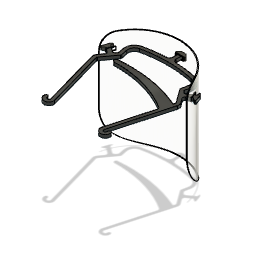
Full_Face_Shield_2 (Autodesk Fusion 360 design; units mm, degrees)
Autodesk Fusion 360 part; units mm, degrees
note: some values were not read from the file. Chosen so that the rebuilt part matches the saved one: which face or edge a step refers to. Set by a fixed rule: which sketch regions a step uses.
sketch "Sketch1" plane through (0, 0, 0) normal (0, 1, 0) x (1, 0, 0)
  line L0 (0, 0) -> (150, 0) construction
  line L1 (150, 0) -> (150, 165) construction
  line L2 (0, 165) -> (0, 0) construction
  line L3 (75, 0) -> (110, 0) construction
  line L4 (75, 0) -> (40, 0) construction
  line L5 (150, 165) -> (150, 115)
  line L6 (0, 165) -> (0, 115) construction
  line L7 (75, 165) -> (15, 165) construction
  line L8 (16.0189, 159.9056) -> (19.5431, 142.2847)
  line L9 (18.5445, 138.1806) -> (1.7256, 117.157)
  line L10 (77.5, 165) -> (135, 165)
  line L11 (133.9811, 159.9056) -> (130.4569, 142.2847)
  line L12 (131.4555, 138.1806) -> (148.2744, 117.157)
  arc A0 (20.1654, 165.8287) -> (16.0189, 159.9056) centre (20.9218, 160.8862) ccw
  arc A1 (133.9811, 159.9056) -> (129.8346, 165.8287) centre (129.0782, 160.8862) ccw
  arc A2 (18.5445, 138.1806) -> (19.5431, 142.2847) centre (14.6402, 141.3041) ccw
  arc A3 (130.4569, 142.2847) -> (131.4555, 138.1806) centre (135.3598, 141.3041) ccw
  arc A4 (1.7256, 117.157) -> (0.9075, 112.391) centre (5.63, 114.0336) ccw
  arc A5 (149.0925, 112.391) -> (148.2744, 117.157) centre (144.37, 114.0336) ccw
  arc A6 (-2.1787, 120.2805) -> (-3.815, 110.7484) centre (5.63, 114.0336) ccw
  line L13 (14.6402, 141.3041) -> (-2.1787, 120.2805)
  line L14 (11.116, 158.925) -> (14.6402, 141.3041)
  arc A7 (19.4091, 170.7711) -> (11.116, 158.925) centre (20.9218, 160.8862) ccw
  arc A8 (130.5909, 170.7711) -> (19.4091, 170.7711) centre (75, -192.5) ccw
  arc A9 (138.884, 158.925) -> (130.5909, 170.7711) centre (129.0782, 160.8862) ccw
  line L15 (138.884, 158.925) -> (135.3598, 141.3041)
  line L16 (135.3598, 141.3041) -> (152.1787, 120.2805)
  arc A10 (153.815, 110.7484) -> (152.1787, 120.2805) centre (144.37, 114.0336) ccw
  line L17 (75, 170) -> (75, 165) construction
  arc A11 (29.827, 93.8884) -> (50.9963, 169.2044) centre (0.8506, 142.666) ccw
  arc A12 (42.1738, 96.8006) -> (56.4371, 169.5244) centre (0.8506, 142.666) ccw
  arc A13 (99.0037, 169.2044) -> (120.173, 93.8884) centre (149.1494, 142.666) ccw
  arc A14 (93.5629, 169.5244) -> (107.8262, 96.8006) centre (149.1494, 142.666) ccw
  circle A15 centre (1.8132, 102.1771) radius 2.5
  circle A16 centre (148.1868, 102.1771) radius 2.5
  line L18 (-3.815, 110.7484) -> (0, 99.7803)
  line L19 (0.9075, 112.391) -> (4.1745, 102.9984)
  line L20 (149.0925, 112.391) -> (145.8255, 102.9984)
  line L21 (153.815, 110.7484) -> (150, 99.7803)
  arc A17 (145.3559, 79.2483) -> (4.6441, 79.2483) centre (75, -70) ccw
  line L22 (-2.88, 72.1259) -> (30, -50)
  arc A18 (30, -50) -> (34.8281, -48.7001) centre (32.414, -49.3501) ccw
  arc A19 (2.5121, 83.771) -> (-2.88, 72.1259) centre (6.7761, 74.7256) ccw
  arc A20 (4.6441, 79.2483) -> (1.948, 73.4257) centre (6.7761, 74.7256) ccw
  line L23 (1.948, 73.4257) -> (34.8281, -48.7001)
  arc A21 (29.827, 93.8884) -> (2.5121, 83.771) centre (75, -70) ccw
  arc A22 (147.4879, 83.771) -> (120.173, 93.8884) centre (75, -70) ccw
  arc A23 (50.9963, 169.2044) -> (20.1654, 165.8287) centre (75, -192.5) ccw
  arc A24 (129.8346, 165.8287) -> (99.0037, 169.2044) centre (75, -192.5) ccw
  line L24 (77.5, 170) -> (77.5, 165)
  line L25 (72.5, 165) -> (72.5, 100)
  line L26 (72.5, 100) -> (72.5, 99.5)
  line L27 (72.5, 99.5) -> (72, 99.5)
  line L28 (72, 99.5) -> (71.8074, 99.5)
  line L29 (77.5, 165) -> (77.5, 99.5)
  line L30 (72.5, 165) -> (72.5, 170.5)
  line L31 (77.5, 169.9914) -> (77.5, 170.5)
  arc A25 (93.5629, 169.5244) -> (77.5, 169.9914) centre (75, -192.5) ccw
  arc A26 (72.5, 169.9914) -> (56.4371, 169.5244) centre (75, -192.5) ccw
  line L32 (150, 165) -> (77.5, 165) construction
  line L33 (75, 165) -> (0, 165) construction
  arc A27 (107.8262, 96.8006) -> (77.5, 99.9816) centre (75, -70) ccw
  arc A28 (72.5, 99.9816) -> (42.1738, 96.8006) centre (75, -70) ccw
  arc A29 (152.88, 72.1259) -> (147.4879, 83.771) centre (143.2239, 74.7256) ccw
  arc A30 (148.052, 73.4257) -> (145.3559, 79.2483) centre (143.2239, 74.7256) ccw
  line L34 (148.052, 73.4257) -> (115.1719, -48.7001)
  line L35 (152.88, 72.1259) -> (120, -50)
  arc A31 (145.3559, 79.2483) -> (4.6441, 79.2483) centre (75, -70) ccw
  arc A32 (115.1719, -48.7001) -> (120, -50) centre (117.586, -49.3501) ccw
  dimension "d1" = 150
  dimension "d2" = 165
  dimension "d3" = 35
  dimension "d4" = 35
  dimension "d5" = 50
  dimension "d6" = 50
  dimension "d7" = 60
  dimension "d8" = 60
  dimension "d9" = 5
  dimension "d14" = 10
  dimension "d15" = -2.5
  constraint horizontal L0
  constraint vertical L1
  constraint horizontal L32
  constraint vertical L2
  constraint coincident L0.start L2.end
  constraint midpoint L0 L3.start
  constraint parallel L0 L3
  constraint parallel L0 L4
  constraint perpendicular L5 L32
  constraint perpendicular L6 L32
  constraint parallel L7 L32
  constraint parallel L10 L32
  constraint coincident L7.end L8
  constraint coincident L7.end A24
  constraint tangent A0 A24
  constraint tangent L8 A0
  constraint coincident L10.end L11
  constraint coincident L10.end A24
  constraint tangent A1 A24
  constraint tangent L11 A1
  constraint equal A0 A1
  constraint tangent L8 A2
  constraint tangent L9 A2
  constraint equal A0 A2
  constraint tangent L11 A3
  constraint tangent L12 A3
  constraint equal A0 A3
  constraint coincident L6.end L9
  constraint coincident L6.end L19
  constraint tangent L9 A4
  constraint tangent A4 L19
  constraint equal A0 A4
  constraint coincident L5.end L12
  constraint coincident L5.end L20
  constraint tangent L12 A5
  constraint tangent A5 L20
  constraint equal A0 A5
  constraint perpendicular L17 L32
  constraint coincident A11.start A22
  constraint coincident A11.end A24
  constraint symmetric L17 A11.end A13.start
  constraint symmetric L17 A11.start A13.end
  constraint symmetric L17 A11 A13
  constraint symmetric L17 A12 A14
  constraint tangent A15 L19
  constraint symmetric L17 A15 A16
  constraint parallel L18 L19
  constraint concentric A4 A6
  constraint parallel L9 L13
  constraint parallel L8 L14
  constraint concentric A0 A7
  constraint concentric A8 A24
  constraint concentric A1 A9
  constraint parallel L11 L15
  constraint parallel L12 L16
  constraint concentric A5 A10
  constraint parallel L20 L21
  constraint tangent A6 L18
  constraint tangent L14 A7
  constraint tangent A7 A8
  constraint tangent A6 L13
  constraint tangent A9 L15
  constraint tangent A8 A9
  constraint tangent L16 A10
  constraint tangent A10 L21
  constraint coincident L2 L18.end
  constraint coincident A15 L19.end
  constraint coincident A16 L20.end
  constraint coincident L1 L21.end
  constraint concentric A17 A22
  constraint tangent A19 A22
  constraint tangent L22 A19
  constraint concentric A11 A12
  constraint concentric A21 A22
  constraint concentric A19 A20
  constraint parallel L22 L23
  constraint tangent A20 L23
  constraint coincident A14.end A22
  constraint concentric A22 A27
  constraint concentric A23 A24
  constraint coincident L17.start A24
  constraint concentric A24 A25
  constraint parallel L25 L26
  constraint perpendicular L26 L27
  constraint perpendicular L26 L28
  constraint perpendicular L27 L29
  constraint parallel L25 L30
  constraint parallel L25 L31
  constraint concentric A25 A26
  constraint coincident L25 A26.start
  constraint collinear L32 L33
  constraint coincident L7.start L32
  constraint coincident L29 A27.end
  constraint coincident L26 A28.start
  constraint concentric A27 A28
  constraint symmetric L17 L22.end L35.end
  constraint symmetric L17 A18.end L34.end
  constraint symmetric L17 L22.start A29.start
  constraint symmetric L17 A19.start A22.start
  constraint symmetric L17 A19 A29
  constraint symmetric L17 A17.end A17.start
  constraint symmetric L17 A20.end A30.start
  constraint symmetric L17 A20 A30
  constraint tangent L35 A32
  measures "d1" distance of L0.start L0.end
  measures "d2" distance of L0.start L2.start
  measures "d3" distance of L3.start L3.end
  measures "d4" distance of L3.start L4.end
  measures "d5" distance of L1.end L5.end
  measures "d6" distance of L2.start L6.end
  measures "d7" distance of L7.start L7.end
  measures "d8" distance of L7.start L10.end
  measures "d9" radius of A0
  measures "d14" radius of A19
sketch "Sketch2" plane through (0, 0, 0) normal (0, 1, 0) x (1, 0, 0)
  arc A0 (74.5, 175.0003) -> (20, 171) centre (74.5, -198.25) ccw
  arc A1 (74.5, 170.0003) -> (20.7301, 166.0536) centre (74.5, -198.25) ccw
  arc A2 (20, 171) -> (11, 159) centre (20.8333, 161) ccw
  line L0 (11, 159) -> (14.1615, 143.4562)
  line L1 (13.1335, 139.2958) -> (-1, 122)
  arc A3 (-1, 122) -> (-3.9689, 110.5533) centre (7.879, 113.5887) ccw
  line L2 (0.3307, 92.0532) -> (30, -50)
  arc A4 (0.3307, 92.0532) -> (-3.9689, 110.5533) centre (-413.7344, 5.5713) ccw
  arc A5 (30, -50) -> (34.8944, -48.9778) centre (32.4472, -49.4889) ccw
  arc A6 (114.1056, -48.9778) -> (119, -50) centre (116.5528, -49.4889) ccw
  arc A7 (13.1335, 139.2958) -> (14.1615, 143.4562) centre (9.2618, 142.4597) ccw
  arc A8 (20.4152, 166.0173) -> (15.8997, 159.9965) centre (20.8333, 161) ccw
  line L3 (15.8997, 159.9965) -> (19.0611, 144.4527)
  arc A9 (17.0052, 136.132) -> (19.0611, 144.4527) centre (9.2618, 142.4597) ccw
  line L4 (17.0052, 136.132) -> (2.7406, 118.6758)
  arc A10 (2.7406, 118.6758) -> (0.8747, 111.7942) centre (7.879, 113.5887) ccw
  arc A11 (5.225, 93.0754) -> (0.8747, 111.7942) centre (-413.7344, 5.5713) ccw
  line L5 (5.225, 93.0754) -> (34.8944, -48.9778)
  line L6 (20.4152, 166.0173) -> (20.7301, 166.0536)
  arc A12 (138, 159) -> (129, 171) centre (128.1667, 161) ccw
  line L7 (133.1003, 159.9965) -> (129.9389, 144.4527)
  line L8 (128.5848, 166.0173) -> (128.2699, 166.0536)
  arc A13 (134.8386, 143.4562) -> (135.8665, 139.2958) centre (139.7382, 142.4597) ccw
  arc A14 (129.9389, 144.4527) -> (131.9948, 136.132) centre (139.7382, 142.4597) ccw
  line L9 (135.8665, 139.2958) -> (150, 122)
  line L10 (138, 159) -> (134.8386, 143.4562)
  arc A15 (129, 171) -> (74.5, 175.0003) centre (74.5, -198.25) ccw
  arc A16 (128.2699, 166.0536) -> (74.5, 170.0003) centre (74.5, -198.25) ccw
  line L11 (131.9948, 136.132) -> (146.2594, 118.6758)
  arc A17 (133.1003, 159.9965) -> (128.5848, 166.0173) centre (128.1667, 161) ccw
  arc A18 (114.1056, -48.9778) -> (119, -50) centre (116.5528, -49.4889) ccw
  arc A19 (148.1253, 111.7942) -> (146.2594, 118.6758) centre (141.121, 113.5887) ccw
  arc A20 (152.9689, 110.5533) -> (148.6693, 92.0532) centre (562.7344, 5.5713) ccw
  line L12 (148.6693, 92.0532) -> (119, -50)
  arc A21 (152.9689, 110.5533) -> (150, 122) centre (141.121, 113.5887) ccw
  arc A22 (141.3302, 87.4373) -> (20, 105) centre (60.9238, -40.1621) ccw
  arc A23 (18.6433, 109.8124) -> (20, 105) centre (19.3216, 107.4062) ccw
  arc A24 (144.5089, 105.6919) -> (38.8673, 114.0893) centre (73.7726, -115.4895) ccw
  arc A25 (143.7795, 100.6741) -> (103.1974, 109.8144) centre (73.7726, -115.4895) ccw
  arc A26 (141.2472, 93.36) -> (103.1974, 109.8144) centre (60.9238, -40.1621) ccw
  arc A27 (38.8673, 114.0893) -> (18.6433, 109.8124) centre (60.9238, -40.1621) ccw
  arc A28 (148.1253, 111.7942) -> (146.9398, 107.0547) centre (562.7344, 5.5713) ccw
  line L13 (142.1794, 85.4361) -> (114.1056, -48.9778)
  arc A29 (144.9419, 98.4876) -> (143.6786, 100.7105) centre (143.0824, 98.9012) ccw
  arc A30 (141.2472, 93.36) -> (144.094, 94.6029) centre (142.2292, 94.9924) ccw
  arc A31 (142.1794, 85.4361) -> (141.3302, 87.4373) centre (140.3146, 85.8256) ccw
  arc A32 (144.5089, 105.6919) -> (146.9398, 107.0547) centre (145.0892, 107.5064) ccw
  line L14 (144.9419, 98.4876) -> (144.094, 94.6029)
  point P0 (149, 0)
  dimension "d17" = -5
  dimension "d18" = 423
  dimension "d19" = -5
  dimension "d20" = 5
  dimension "d23" = 1.905
  dimension "d24" = 1.905
  dimension "d25" = 1.905
  constraint tangent A2 L0
  constraint tangent A3 A4
  constraint tangent L2 A4
  constraint tangent A5 L5
  constraint tangent A22 A23
  constraint concentric A22 A26
  constraint coincident A24.end A26
  constraint concentric A24 A25
  constraint concentric A26 A27
  constraint tangent A26 A30
  constraint equal A29 A30
  constraint tangent A22 A31
  constraint tangent L13 A31
  constraint tangent A24 A32
  constraint tangent A28 A32
  constraint coincident A29 A25.start
  measures "d18" radius of A4
  measures "d20" radius of A7
  measures "d23" radius of A29
  measures "d24" radius of A31
  measures "d25" radius of A32
sketch "Sketch3" plane through (0, 0, 0) normal (0, 1, 0) x (1, 0, 0)
  arc A0 (143.1611, 90.1462) -> (22.4815, 123.2089) centre (28.0682, -93.1729) ccw
  arc A1 (151.4699, 109.6951) -> (21.7483, 130.6442) centre (45.713, -133.0677) ccw
  line L0 (15.076, 155.7601) -> (17.5617, 143.3317)
  line L1 (17.1252, 141.3396) -> (-1.8602, 115.2347)
  line L2 (-2.2518, 113.0551) -> (50.8, -76.2)
  line L3 (75.1061, 175.0001) -> (75.1061, 157.48) construction
  line L4 (135.1363, 155.7601) -> (132.6506, 143.3317)
  line L5 (133.0871, 141.3396) -> (152.0341, 115.2875)
  arc A2 (125.4227, 170.6518) -> (24.7896, 170.6518) centre (75.1061, -57.0962) ccw
  arc A3 (24.7896, 170.6518) -> (15.076, 155.7601) centre (27.5294, 158.2508) ccw
  arc A4 (135.1363, 155.7601) -> (125.4227, 170.6518) centre (122.6829, 158.2508) ccw
  arc A5 (17.1252, 141.3396) -> (17.5617, 143.3317) centre (15.071, 142.8336) ccw
  arc A6 (132.6506, 143.3317) -> (133.0871, 141.3396) centre (135.1413, 142.8336) ccw
  arc A7 (-1.8602, 115.2347) -> (-2.2518, 113.0551) centre (0.1939, 113.7407) ccw
  arc A8 (152.4258, 113.1086) -> (152.0341, 115.2875) centre (149.9799, 113.7935) ccw
  line L6 (-8.3661, 111.3412) -> (44.6857, -77.914)
  arc A9 (-6.9957, 118.9696) -> (-8.3661, 111.3412) centre (0.1939, 113.7407) ccw
  line L7 (8.8493, 154.5148) -> (11.0075, 143.7239)
  arc A10 (23.4197, 176.8522) -> (8.8493, 154.5148) centre (27.5294, 158.2508) ccw
  arc A11 (126.7925, 176.8522) -> (23.4197, 176.8522) centre (75.1061, -57.0962) ccw
  arc A12 (141.363, 154.5148) -> (126.7925, 176.8522) centre (122.6829, 158.2508) ccw
  line L8 (141.363, 154.5148) -> (139.2048, 143.7239)
  arc A13 (158.5406, 111.3962) -> (157.1696, 119.0224) centre (149.9799, 113.7935) ccw
  line L9 (158.5406, 111.3962) -> (105.527, -77.9124)
  arc A14 (99.4123, -76.2) -> (105.527, -77.9124) centre (102.4696, -77.0562) ccw
  arc A15 (44.6857, -77.914) -> (50.8, -76.2) centre (47.7428, -77.057) ccw
  line L10 (152.4258, 113.1086) -> (151.4699, 109.6951)
  line L11 (144.8041, 85.892) -> (99.4123, -76.2)
  arc A16 (10.3842, 0.0056) -> (29.4342, 0.0197) centre (19.9103, -1.4524) ccw
  arc A17 (16.6611, -0.9551) -> (23.1587, -0.9503) centre (19.9103, -1.4524) ccw
  arc A18 (16.6611, -0.9551) -> (10.3842, 0.0056) centre (13.5226, -0.4747) ccw
  arc A19 (120.7781, 0.0197) -> (139.8281, 0.0056) centre (130.302, -1.4524) ccw
  arc A20 (127.0535, -0.9503) -> (133.5512, -0.9551) centre (130.302, -1.4524) ccw
  arc A21 (139.8281, 0.0056) -> (133.5512, -0.9551) centre (136.6896, -0.4747) ccw
  line L12 (120.7781, 0.0197) -> (120.8502, 0.3539)
  line L13 (-13.4671, 150.4121) -> (-17.879, 137.4466)
  line L14 (-1.0754, 133.5877) -> (-10.7402, 140.6166)
  line L15 (-12.1427, 135.7823) -> (-10.7402, 140.6166)
  line L16 (3.1554, 139.4051) -> (-10.0906, 149.0386)
  line L17 (-8.5671, 153.5158) -> (-10.0906, 149.0386)
  line L18 (-17.879, 137.4466) -> (-12.1427, 135.7823)
  line L19 (-8.5671, 153.5158) -> (-10.2135, 154.0761)
  line L20 (11.0075, 143.7239) -> (8.4776, 140.2454)
  line L21 (-0.2351, 128.2655) -> (-6.9957, 118.9696)
  arc A22 (-0.2351, 128.2655) -> (-1.0754, 133.5877) centre (-3.3163, 130.5064) ccw
  arc A23 (3.1554, 139.4051) -> (8.4776, 140.2454) centre (5.3964, 142.4864) ccw
  line L22 (-8.5671, 153.5158) -> (-10.2135, 154.0761)
  line L23 (-10.2135, 154.0761) -> (-13.4671, 150.4121)
  arc A24 (23.3191, 130.7822) -> (23.4173, 123.231) centre (22.86, 127) ccw
  arc A25 (141.7346, 140.2454) -> (147.0568, 139.4051) centre (144.8159, 142.4864) ccw
  arc A26 (151.2877, 133.5877) -> (150.4473, 128.2655) centre (153.5286, 130.5064) ccw
  line L24 (151.2877, 133.5877) -> (160.9524, 140.6166)
  line L25 (147.0568, 139.4051) -> (160.3029, 149.0386)
  line L26 (158.7794, 153.5158) -> (160.3029, 149.0386)
  line L27 (168.0912, 137.4466) -> (162.355, 135.7823)
  line L28 (163.6794, 150.4121) -> (168.0912, 137.4466)
  line L29 (162.355, 135.7823) -> (160.9524, 140.6166)
  line L30 (160.4258, 154.0761) -> (163.6794, 150.4121)
  line L31 (158.7794, 153.5158) -> (160.4258, 154.0761)
  line L32 (139.2048, 143.7239) -> (141.7346, 140.2454)
  line L33 (150.4473, 128.2655) -> (157.1696, 119.0224)
  arc A27 (144.8041, 85.892) -> (143.1611, 90.1462) centre (141.1353, 86.9194) ccw
  dimension "d26" = 7.62
  dimension "d27" = 12.7
  dimension "d28" = 2.54
  dimension "d32" = 19.05
  dimension "d33" = -6.35
  dimension "d41" = 3.81
  dimension "d42" = 3.81
  constraint coincident A0.end A24
  constraint coincident A1.end A24
  constraint vertical L3
  constraint symmetric L2.end L3 A14.start
  constraint tangent A2 A3
  constraint tangent L0 A3
  constraint tangent A2 A4
  constraint tangent L4 A4
  constraint equal A3 A4
  constraint tangent L0 A5
  constraint tangent L1 A5
  constraint tangent L4 A6
  constraint tangent L5 A6
  constraint equal A5 A6
  constraint tangent L1 A7
  constraint tangent L2 A7
  constraint equal A5 A7
  constraint tangent L5 A8
  constraint tangent A8 L10
  constraint equal A5 A8
  constraint tangent L2 A15
  constraint collinear L10 L11
  constraint parallel L2 L6
  constraint concentric A7 A9
  constraint parallel L1 L20
  constraint parallel L0 L7
  constraint concentric A3 A10
  constraint concentric A2 A11
  constraint concentric A4 A12
  constraint parallel L4 L8
  constraint parallel L5 L32
  constraint concentric A8 A13
  constraint tangent L7 A10
  constraint tangent A10 A11
  constraint tangent A13 L9
  constraint tangent A11 A12
  constraint tangent A12 L8
  constraint tangent A13 L32
  constraint coincident L2 A16.end
  constraint tangent A17 A18
  constraint symmetric L3 A16.end A19.start
  constraint symmetric L3 A16.start A19.end
  constraint symmetric L3 A16 A19
  constraint symmetric L3 A17.end A20.start
  constraint symmetric L3 A17.start A20.end
  constraint symmetric L3 A17 A20
  constraint symmetric L3 A18 A21
  constraint coincident L11 L12.end
  constraint perpendicular L14 L20
  constraint perpendicular L16 L20
  constraint parallel L13 L17
  constraint perpendicular L15 L18
  constraint perpendicular L17 L19
  constraint collinear L20 L21
  constraint tangent L21 A22
  constraint tangent L14 A22
  constraint tangent L16 A23
  constraint tangent L20 A23
  constraint equal A22 A23
  constraint coincident A0 A24.end
  constraint coincident A1 A24.start
  constraint symmetric L3 L17.start L26.start
  constraint symmetric L3 L13.end L27.start
  constraint symmetric L3 L14.end L24.end
  constraint symmetric L3 L16.end L25.end
  constraint symmetric L3 L15.start L27.end
  constraint symmetric L3 L21.start A26.end
  constraint symmetric L3 L14.start A26.start
  constraint symmetric L3 A22 A26
  constraint symmetric L3 L16.start A25.end
  constraint symmetric L3 L20.end A25.start
  constraint symmetric L3 A23 A25
  constraint symmetric L3 L19.end L30.start
  constraint symmetric L3 L13.start L28.start
  constraint collinear L32 L33
  constraint tangent A0 A27
  constraint tangent L11 A27
  measures "d26" diameter of A24
  measures "d27" radius of A3
  measures "d28" radius of A5
  measures "d32" distance of A16.end A16.start
  measures "d41" radius of A22
  measures "d42" radius of A27
extrude "Extrude1" add sketch "Sketch3" along normal blind 6.223 contours A0 A1 L0 L1 L2 L4 L5 A2 A3 A4 A5 A6 A7 A8 L6 A9 L7 A10 A11 A12 L8 A13 L9 L10 L11 A16 A19 L12 L13 L14 L15 L16 L17 L18 L19 L20 L21 A22 A23 L22 L23 A24 A25 A26 L24 L25 L26 L27 L28 L29 L30 L31 L32 L33 A27 | A1 A24 makes body 1
sketch "Sketch4" plane through (0, 6.223, 0) normal (0, 1, 0) x (-1, 0, 0)
  arc A0 (-143.1611, -90.1462) -> (-22.4815, -123.2089) centre (-28.0682, 93.1729) ccw
  line L0 (-144.8041, -85.892) -> (-120.8502, -0.3539)
  line L1 (-124.7356, 9.3193) -> (-158.5406, -111.3962)
  arc A1 (-158.5406, -111.3962) -> (-157.1696, -119.0224) centre (-149.9799, -113.7935) ccw
  line L2 (-157.1696, -119.0224) -> (-150.4473, -128.2655)
  line L3 (-139.2048, -143.7239) -> (-141.363, -154.5148)
  arc A2 (-141.363, -154.5148) -> (-126.7925, -176.8522) centre (-122.6829, -158.2508) ccw
  arc A3 (-126.7925, -176.8522) -> (-23.4197, -176.8522) centre (-75.1061, 57.0962) ccw
  arc A4 (-23.4197, -176.8522) -> (-8.8493, -154.5148) centre (-27.5294, -158.2508) ccw
  line L4 (-8.8493, -154.5148) -> (-11.0075, -143.7239)
  line L5 (-11.0075, -143.7239) -> (-8.4776, -140.2454)
  arc A5 (6.9957, -118.9696) -> (8.3661, -111.3412) centre (-0.1939, -113.7407) ccw
  line L6 (8.3661, -111.3412) -> (-25.4605, 9.3307)
  line L7 (-29.4342, -0.0197) -> (2.2518, -113.0551)
  arc A6 (1.8602, -115.2347) -> (2.2518, -113.0551) centre (-0.1939, -113.7407) ccw
  line L8 (1.8602, -115.2347) -> (-17.1252, -141.3396)
  arc A7 (-17.1252, -141.3396) -> (-17.5617, -143.3317) centre (-15.071, -142.8336) ccw
  line L9 (-17.5617, -143.3317) -> (-15.076, -155.7601)
  arc A8 (-24.7896, -170.6518) -> (-15.076, -155.7601) centre (-27.5294, -158.2508) ccw
  arc A9 (-125.4227, -170.6518) -> (-24.7896, -170.6518) centre (-75.1061, 57.0962) ccw
  arc A10 (-135.1363, -155.7601) -> (-125.4227, -170.6518) centre (-122.6829, -158.2508) ccw
  line L10 (-135.1363, -155.7601) -> (-132.6506, -143.3317)
  arc A11 (-132.6506, -143.3317) -> (-133.0871, -141.3396) centre (-135.1413, -142.8336) ccw
  line L11 (-133.0871, -141.3396) -> (-152.0341, -115.2875)
  arc A12 (-152.4258, -113.1086) -> (-152.0341, -115.2875) centre (-149.9799, -113.7935) ccw
  line L12 (-152.4258, -113.1086) -> (-151.4699, -109.6951)
  arc A13 (-151.4699, -109.6951) -> (-23.3191, -130.7822) centre (-45.713, 133.0677) ccw
  arc A14 (-23.3191, -130.7822) -> (-22.4815, -123.2089) centre (-22.86, -127) ccw
  arc A15 (-144.8041, -85.892) -> (-143.1611, -90.1462) centre (-141.1353, -86.9194) ccw
  line L13 (-120.8502, -0.3539) -> (-120.7781, -0.0197)
  arc A16 (-120.7781, -0.0197) -> (-124.7356, 9.3193) centre (-130.302, 1.4524) ccw
  arc A17 (-151.2877, -133.5877) -> (-150.4473, -128.2655) centre (-153.5286, -130.5064) ccw
  line L14 (-151.2877, -133.5877) -> (-160.9524, -140.6166)
  line L15 (-160.9524, -140.6166) -> (-162.355, -135.7823)
  line L16 (-162.355, -135.7823) -> (-168.0912, -137.4466)
  line L17 (-168.0912, -137.4466) -> (-163.6794, -150.4121)
  line L18 (-163.6794, -150.4121) -> (-160.4258, -154.0761)
  line L19 (-160.4258, -154.0761) -> (-158.7794, -153.5158)
  line L20 (-158.7794, -153.5158) -> (-160.3029, -149.0386)
  line L21 (-160.3029, -149.0386) -> (-147.0568, -139.4051)
  arc A18 (-141.7346, -140.2454) -> (-147.0568, -139.4051) centre (-144.8159, -142.4864) ccw
  line L22 (-141.7346, -140.2454) -> (-139.2048, -143.7239)
  arc A19 (-3.1554, -139.4051) -> (-8.4776, -140.2454) centre (-5.3964, -142.4864) ccw
  line L23 (-3.1554, -139.4051) -> (10.0906, -149.0386)
  line L24 (10.0906, -149.0386) -> (8.5671, -153.5158)
  line L25 (8.5671, -153.5158) -> (10.2135, -154.0761)
  line L26 (10.2135, -154.0761) -> (13.4671, -150.4121)
  line L27 (13.4671, -150.4121) -> (17.879, -137.4466)
  line L28 (17.879, -137.4466) -> (12.1427, -135.7823)
  line L29 (12.1427, -135.7823) -> (10.7402, -140.6166)
  line L30 (10.7402, -140.6166) -> (1.0754, -133.5877)
  arc A20 (0.2351, -128.2655) -> (1.0754, -133.5877) centre (3.3163, -130.5064) ccw
  line L31 (0.2351, -128.2655) -> (6.9957, -118.9696)
  arc A21 (-25.4605, 9.3307) -> (-29.4342, -0.0197) centre (-19.9103, 1.4524) ccw
sketch "Sketch6" plane through (0, 6.223, 0) normal (0, 1, 0) x (-1, 0, 0)
sketch "Sketch7" plane through (0, 0, 0) normal (0, 1, 0) x (1, 0, 0)
extrude "Extrude2" add sketch "Sketch3" along normal blind 6.096 separate body contours A0 A1 L0 L1 L2 L4 L5 A2 A3 A4 A5 A6 A7 A8 L6 A9 L7 A10 A11 A12 L8 A13 L9 L10 L11 A16 A19 L12 L13 L14 L15 L16 L17 L18 L19 L20 L21 A22 A23 L22 L23 A24 A25 A26 L24 L25 L26 L27 L28 L29 L30 L31 L32 L33 A27 | L9 A19 A20 A21 | L6 A16 A17 A18 makes body 2
sketch "Sketch8" plane through (0, 0, 0) normal (0, -1, 0) x (1, 0, 0)
  arc A0 (139.8281, -0.0056) -> (120.7781, -0.0197) centre (130.302, 1.4524) ccw
  line L0 (120.7781, -0.0197) -> (120.8502, -0.3539)
  line L1 (120.8502, -0.3539) -> (144.8041, -85.892)
  arc A1 (22.4815, -123.2089) -> (143.1611, -90.1462) centre (28.0682, 93.1729) ccw
  arc A2 (22.4815, -123.2089) -> (21.7483, -130.6442) centre (22.86, -127) ccw
  arc A3 (21.7483, -130.6442) -> (151.4699, -109.6951) centre (45.713, 133.0677) ccw
  line L2 (151.4699, -109.6951) -> (152.4258, -113.1086)
  arc A4 (152.0341, -115.2875) -> (152.4258, -113.1086) centre (149.9799, -113.7935) ccw
  line L3 (152.0341, -115.2875) -> (133.0871, -141.3396)
  arc A5 (133.0871, -141.3396) -> (132.6506, -143.3317) centre (135.1413, -142.8336) ccw
  line L4 (132.6506, -143.3317) -> (135.1363, -155.7601)
  arc A6 (125.4227, -170.6518) -> (135.1363, -155.7601) centre (122.6829, -158.2508) ccw
  arc A7 (24.7896, -170.6518) -> (125.4227, -170.6518) centre (75.1061, 57.0962) ccw
  arc A8 (15.076, -155.7601) -> (24.7896, -170.6518) centre (27.5294, -158.2508) ccw
  line L5 (15.076, -155.7601) -> (17.5617, -143.3317)
  arc A9 (17.5617, -143.3317) -> (17.1252, -141.3396) centre (15.071, -142.8336) ccw
  line L6 (17.1252, -141.3396) -> (-1.8602, -115.2347)
  arc A10 (-2.2518, -113.0551) -> (-1.8602, -115.2347) centre (0.1939, -113.7407) ccw
  line L7 (-2.2518, -113.0551) -> (29.4342, -0.0197)
  arc A11 (29.4342, -0.0197) -> (10.3842, -0.0056) centre (19.9103, 1.4524) ccw
  arc A12 (10.3842, -0.0056) -> (16.6611, 0.9551) centre (13.5226, 0.4747) ccw
  arc A13 (23.1898, 1.2301) -> (16.6611, 0.9551) centre (19.9103, 1.4524) ccw
  line L8 (23.1898, 1.2301) -> (-8.3661, -111.3412)
  arc A14 (-8.3661, -111.3412) -> (-6.9957, -118.9696) centre (0.1939, -113.7407) ccw
  line L9 (-6.9957, -118.9696) -> (-0.2351, -128.2655)
  line L10 (11.0075, -143.7239) -> (8.8493, -154.5148)
  arc A15 (8.8493, -154.5148) -> (23.4197, -176.8522) centre (27.5294, -158.2508) ccw
  arc A16 (23.4197, -176.8522) -> (126.7925, -176.8522) centre (75.1061, 57.0962) ccw
  arc A17 (126.7925, -176.8522) -> (141.363, -154.5148) centre (122.6829, -158.2508) ccw
  line L11 (141.363, -154.5148) -> (139.2048, -143.7239)
  line L12 (139.2048, -143.7239) -> (141.7346, -140.2454)
  arc A18 (157.1696, -119.0224) -> (158.5406, -111.3962) centre (149.9799, -113.7935) ccw
  line L13 (158.5406, -111.3962) -> (127.0318, 1.1197)
  arc A19 (133.5512, 0.9551) -> (127.0318, 1.1197) centre (130.302, 1.4524) ccw
  arc A20 (133.5512, 0.9551) -> (139.8281, -0.0056) centre (136.6896, 0.4747) ccw
  arc A21 (143.1611, -90.1462) -> (144.8041, -85.892) centre (141.1353, -86.9194) ccw
  arc A22 (-1.0754, -133.5877) -> (-0.2351, -128.2655) centre (-3.3163, -130.5064) ccw
  line L14 (-1.0754, -133.5877) -> (-10.7402, -140.6166)
  line L15 (-10.7402, -140.6166) -> (-12.1427, -135.7823)
  line L16 (-12.1427, -135.7823) -> (-17.879, -137.4466)
  line L17 (-17.879, -137.4466) -> (-13.4671, -150.4121)
  line L18 (-13.4671, -150.4121) -> (-10.2135, -154.0761)
  line L19 (-10.2135, -154.0761) -> (-8.5671, -153.5158)
  line L20 (-8.5671, -153.5158) -> (-10.0906, -149.0386)
  line L21 (-10.0906, -149.0386) -> (3.1554, -139.4051)
  arc A23 (8.4776, -140.2454) -> (3.1554, -139.4051) centre (5.3964, -142.4864) ccw
  line L22 (8.4776, -140.2454) -> (11.0075, -143.7239)
  arc A24 (147.0568, -139.4051) -> (141.7346, -140.2454) centre (144.8159, -142.4864) ccw
  line L23 (147.0568, -139.4051) -> (160.3029, -149.0386)
  line L24 (160.3029, -149.0386) -> (158.7794, -153.5158)
  line L25 (158.7794, -153.5158) -> (160.4258, -154.0761)
  line L26 (160.4258, -154.0761) -> (163.6794, -150.4121)
  line L27 (163.6794, -150.4121) -> (168.0912, -137.4466)
  line L28 (168.0912, -137.4466) -> (162.355, -135.7823)
  line L29 (162.355, -135.7823) -> (160.9524, -140.6166)
  line L30 (160.9524, -140.6166) -> (151.2877, -133.5877)
  arc A25 (150.4473, -128.2655) -> (151.2877, -133.5877) centre (153.5286, -130.5064) ccw
  line L31 (150.4473, -128.2655) -> (157.1696, -119.0224)
sketch "Sketch9" plane through (0, 0, 0) normal (0, -1, 0) x (1, 0, 0)
sketch "Sketch10" plane through (0, 0, 0) normal (0, -1, 0) x (1, 0, 0)
  arc A0 (139.8281, -0.0056) -> (120.7781, -0.0197) centre (130.302, 1.4524) ccw
  line L0 (120.7781, -0.0197) -> (120.8502, -0.3539)
  line L1 (120.8502, -0.3539) -> (144.8041, -85.892)
  arc A1 (143.1611, -90.1462) -> (144.8041, -85.892) centre (141.1353, -86.9194) ccw
  arc A2 (22.4815, -123.2089) -> (143.1611, -90.1462) centre (28.0682, 93.1729) ccw
  arc A3 (22.4815, -123.2089) -> (21.7483, -130.6442) centre (22.86, -127) ccw
  arc A4 (21.7483, -130.6442) -> (151.4699, -109.6951) centre (45.713, 133.0677) ccw
  line L2 (151.4699, -109.6951) -> (152.4258, -113.1086)
  arc A5 (152.0341, -115.2875) -> (152.4258, -113.1086) centre (149.9799, -113.7935) ccw
  line L3 (152.0341, -115.2875) -> (133.0871, -141.3396)
  arc A6 (133.0871, -141.3396) -> (132.6506, -143.3317) centre (135.1413, -142.8336) ccw
  line L4 (132.6506, -143.3317) -> (135.1363, -155.7601)
  arc A7 (125.4227, -170.6518) -> (135.1363, -155.7601) centre (122.6829, -158.2508) ccw
  arc A8 (24.7896, -170.6518) -> (125.4227, -170.6518) centre (75.1061, 57.0962) ccw
  arc A9 (15.076, -155.7601) -> (24.7896, -170.6518) centre (27.5294, -158.2508) ccw
  line L5 (15.076, -155.7601) -> (17.5617, -143.3317)
  arc A10 (17.5617, -143.3317) -> (17.1252, -141.3396) centre (15.071, -142.8336) ccw
  line L6 (17.1252, -141.3396) -> (-1.8602, -115.2347)
  arc A11 (-2.2518, -113.0551) -> (-1.8602, -115.2347) centre (0.1939, -113.7407) ccw
  line L7 (-2.2518, -113.0551) -> (29.4342, -0.0197)
  arc A12 (29.4342, -0.0197) -> (10.3842, -0.0056) centre (19.9103, 1.4524) ccw
  arc A13 (10.3842, -0.0056) -> (16.6611, 0.9551) centre (13.5226, 0.4747) ccw
  arc A14 (23.1898, 1.2301) -> (16.6611, 0.9551) centre (19.9103, 1.4524) ccw
  line L8 (23.1898, 1.2301) -> (-8.3661, -111.3412)
  arc A15 (-8.3661, -111.3412) -> (-6.9957, -118.9696) centre (0.1939, -113.7407) ccw
  line L9 (-6.9957, -118.9696) -> (-0.2351, -128.2655)
  arc A16 (-1.0754, -133.5877) -> (-0.2351, -128.2655) centre (-3.3163, -130.5064) ccw
  line L10 (-1.0754, -133.5877) -> (-10.7402, -140.6166)
  line L11 (-10.7402, -140.6166) -> (-12.1427, -135.7823)
  line L12 (-12.1427, -135.7823) -> (-17.879, -137.4466)
  line L13 (-17.879, -137.4466) -> (-13.4671, -150.4121)
  line L14 (-13.4671, -150.4121) -> (-10.2135, -154.0761)
  line L15 (-10.2135, -154.0761) -> (-8.5671, -153.5158)
  line L16 (-8.5671, -153.5158) -> (-10.0906, -149.0386)
  line L17 (-10.0906, -149.0386) -> (3.1554, -139.4051)
  arc A17 (8.4776, -140.2454) -> (3.1554, -139.4051) centre (5.3964, -142.4864) ccw
  line L18 (8.4776, -140.2454) -> (11.0075, -143.7239)
  line L19 (11.0075, -143.7239) -> (8.8493, -154.5148)
  arc A18 (8.8493, -154.5148) -> (23.4197, -176.8522) centre (27.5294, -158.2508) ccw
  arc A19 (23.4197, -176.8522) -> (126.7925, -176.8522) centre (75.1061, 57.0962) ccw
  arc A20 (126.7925, -176.8522) -> (141.363, -154.5148) centre (122.6829, -158.2508) ccw
  line L20 (141.363, -154.5148) -> (139.2048, -143.7239)
  line L21 (139.2048, -143.7239) -> (141.7346, -140.2454)
  arc A21 (147.0568, -139.4051) -> (141.7346, -140.2454) centre (144.8159, -142.4864) ccw
  line L22 (147.0568, -139.4051) -> (160.3029, -149.0386)
  line L23 (160.3029, -149.0386) -> (158.7794, -153.5158)
  line L24 (158.7794, -153.5158) -> (160.4258, -154.0761)
  line L25 (160.4258, -154.0761) -> (163.6794, -150.4121)
  line L26 (163.6794, -150.4121) -> (168.0912, -137.4466)
  line L27 (168.0912, -137.4466) -> (162.355, -135.7823)
  line L28 (162.355, -135.7823) -> (160.9524, -140.6166)
  line L29 (160.9524, -140.6166) -> (151.2877, -133.5877)
  arc A22 (150.4473, -128.2655) -> (151.2877, -133.5877) centre (153.5286, -130.5064) ccw
  line L30 (150.4473, -128.2655) -> (157.1696, -119.0224)
  arc A23 (157.1696, -119.0224) -> (158.5406, -111.3962) centre (149.9799, -113.7935) ccw
  line L31 (158.5406, -111.3962) -> (127.0318, 1.1197)
  arc A24 (133.5512, 0.9551) -> (127.0318, 1.1197) centre (130.302, 1.4524) ccw
  arc A25 (133.5512, 0.9551) -> (139.8281, -0.0056) centre (136.6896, 0.4747) ccw
chamfer "Chamfer1" distance 3.81 angle 45 1 edges at (-12.1427, 3.048, -135.7823) on bodies 2
chamfer "Chamfer2" distance 3.81 angle 45 1 edges at (162.355, 3.048, -135.7823) on bodies 2
sketch "Sketch11" plane through (0, 0, 0) normal (0, 0, 1) x (1, 0, 0)
sketch "Sketch12" plane through (0, 6.096, 0) normal (0, 1, 0) x (-1, 0, 0)
  line L0 (-161.2934, -139.4414) -> (-166.0141, -136.844)
  line L1 (-166.0141, -136.844) -> (-168.0912, -137.4466)
  line L2 (-168.0912, -137.4466) -> (-163.6794, -150.4121)
  line L3 (-163.6794, -150.4121) -> (-160.4258, -154.0761)
  line L4 (-160.4258, -154.0761) -> (-158.7794, -153.5158)
  line L5 (-158.7794, -153.5158) -> (-160.3029, -149.0386)
  line L6 (-160.3029, -149.0386) -> (-147.0568, -139.4051)
  arc A0 (-141.7346, -140.2454) -> (-147.0568, -139.4051) centre (-144.8159, -142.4864) ccw
  line L7 (-141.7346, -140.2454) -> (-139.2048, -143.7239)
  line L8 (-139.2048, -143.7239) -> (-141.363, -154.5148)
  arc A1 (-141.363, -154.5148) -> (-126.7925, -176.8522) centre (-122.6829, -158.2508) ccw
  arc A2 (-126.7925, -176.8522) -> (-23.4197, -176.8522) centre (-75.1061, 57.0962) ccw
  arc A3 (-23.4197, -176.8522) -> (-8.8493, -154.5148) centre (-27.5294, -158.2508) ccw
  line L9 (-8.8493, -154.5148) -> (-11.0075, -143.7239)
  line L10 (-11.0075, -143.7239) -> (-8.4776, -140.2454)
  arc A4 (-3.1554, -139.4051) -> (-8.4776, -140.2454) centre (-5.3964, -142.4864) ccw
  line L11 (-3.1554, -139.4051) -> (10.0906, -149.0386)
  line L12 (10.0906, -149.0386) -> (8.5671, -153.5158)
  line L13 (8.5671, -153.5158) -> (10.2135, -154.0761)
  line L14 (10.2135, -154.0761) -> (13.4671, -150.4121)
  line L15 (13.4671, -150.4121) -> (17.879, -137.4466)
  line L16 (17.879, -137.4466) -> (15.8018, -136.844)
  line L17 (15.8018, -136.844) -> (11.0811, -139.4414)
  line L18 (11.0811, -139.4414) -> (10.7402, -140.6166)
  line L19 (10.7402, -140.6166) -> (1.0754, -133.5877)
  arc A5 (0.2351, -128.2655) -> (1.0754, -133.5877) centre (3.3163, -130.5064) ccw
  line L20 (0.2351, -128.2655) -> (6.9957, -118.9696)
  arc A6 (6.9957, -118.9696) -> (8.3661, -111.3412) centre (-0.1939, -113.7407) ccw
  line L21 (8.3661, -111.3412) -> (-23.1898, 1.2301)
  arc A7 (-16.6611, 0.9551) -> (-23.1898, 1.2301) centre (-19.9103, 1.4524) ccw
  arc A8 (-16.6611, 0.9551) -> (-10.3842, -0.0056) centre (-13.5226, 0.4747) ccw
  arc A9 (-10.3842, -0.0056) -> (-29.4342, -0.0197) centre (-19.9103, 1.4524) ccw
  line L22 (-29.4342, -0.0197) -> (2.2518, -113.0551)
  arc A10 (1.8602, -115.2347) -> (2.2518, -113.0551) centre (-0.1939, -113.7407) ccw
  line L23 (1.8602, -115.2347) -> (-17.1252, -141.3396)
  arc A11 (-17.1252, -141.3396) -> (-17.5617, -143.3317) centre (-15.071, -142.8336) ccw
  line L24 (-17.5617, -143.3317) -> (-15.076, -155.7601)
  arc A12 (-24.7896, -170.6518) -> (-15.076, -155.7601) centre (-27.5294, -158.2508) ccw
  arc A13 (-125.4227, -170.6518) -> (-24.7896, -170.6518) centre (-75.1061, 57.0962) ccw
  arc A14 (-135.1363, -155.7601) -> (-125.4227, -170.6518) centre (-122.6829, -158.2508) ccw
  line L25 (-135.1363, -155.7601) -> (-132.6506, -143.3317)
  arc A15 (-132.6506, -143.3317) -> (-133.0871, -141.3396) centre (-135.1413, -142.8336) ccw
  line L26 (-133.0871, -141.3396) -> (-152.0341, -115.2875)
  arc A16 (-152.4258, -113.1086) -> (-152.0341, -115.2875) centre (-149.9799, -113.7935) ccw
  line L27 (-152.4258, -113.1086) -> (-151.4699, -109.6951)
  arc A17 (-151.4699, -109.6951) -> (-21.7483, -130.6442) centre (-45.713, 133.0677) ccw
  arc A18 (-21.7483, -130.6442) -> (-22.4815, -123.2089) centre (-22.86, -127) ccw
  arc A19 (-143.1611, -90.1462) -> (-22.4815, -123.2089) centre (-28.0682, 93.1729) ccw
  arc A20 (-144.8041, -85.892) -> (-143.1611, -90.1462) centre (-141.1353, -86.9194) ccw
  line L28 (-144.8041, -85.892) -> (-120.8502, -0.3539)
  line L29 (-120.8502, -0.3539) -> (-120.7781, -0.0197)
  arc A21 (-120.7781, -0.0197) -> (-139.8281, -0.0056) centre (-130.302, 1.4524) ccw
  arc A22 (-139.8281, -0.0056) -> (-133.5512, 0.9551) centre (-136.6896, 0.4747) ccw
  arc A23 (-127.0318, 1.1197) -> (-133.5512, 0.9551) centre (-130.302, 1.4524) ccw
  line L30 (-127.0318, 1.1197) -> (-158.5406, -111.3962)
  arc A24 (-158.5406, -111.3962) -> (-157.1696, -119.0224) centre (-149.9799, -113.7935) ccw
  line L31 (-157.1696, -119.0224) -> (-150.4473, -128.2655)
  arc A25 (-151.2877, -133.5877) -> (-150.4473, -128.2655) centre (-153.5286, -130.5064) ccw
  line L32 (-151.2877, -133.5877) -> (-160.9524, -140.6166)
  line L33 (-160.9524, -140.6166) -> (-161.2934, -139.4414)
  arc A26 (-160.02, -127) -> (10.16, -127) centre (-74.93, -111.76) ccw
  arc A27 (-161.5826, -127.2799) -> (11.7226, -127.2799) centre (-74.93, -111.76) ccw
  line L34 (11.7226, -127.2799) -> (10.16, -127)
  line L35 (-160.02, -127) -> (-161.5826, -127.2799)
  dimension "d45" = 1.5875
extrude "Extrude3" add sketch "Sketch12" along normal blind 25.4 and the other way blind 177.8 separate body contours L32 A26 A27 L35 | L6 L32 A26 A27 | L6 L11 A26 A27 | L11 L19 A26 A27 | L19 A26 A27 L34 makes body 3
sketch "Sketch13" plane through (0, 0, 0) normal (1, 0, 0) x (0, 0, -1)
  arc A0 (127, -88.9) -> (203.2, -165.1) centre (204.8972, -87.2028) ccw
  line L0 (127, -88.9) -> (114.3, -88.9)
  line L1 (114.3, -88.9) -> (114.3, -177.8)
  line L2 (114.3, -177.8) -> (203.2, -177.8)
  line L3 (203.2, -177.8) -> (203.2, -165.1)
  constraint horizontal L0
  constraint perpendicular L0 L1
  constraint perpendicular L1 L2
extrude "Extrude4" cut sketch "Sketch13" along normal blind -50.8 and the other way blind -292.1 bodies 3
fillet "Fillet1" radius 25.4 2 edges at (-10.9413, 31.496, -127.1399) (160.8013, 31.496, -127.1399) on bodies 3
sketch "Sketch14" plane through (0, 6.096, 0) normal (0, 1, 0) x (-1, 0, 0)
  line L0 (-161.2934, -139.4414) -> (-166.0141, -136.844)
  line L1 (-166.0141, -136.844) -> (-168.0912, -137.4466)
  line L2 (-168.0912, -137.4466) -> (-163.6794, -150.4121)
  line L3 (-163.6794, -150.4121) -> (-160.4258, -154.0761)
  line L4 (-160.4258, -154.0761) -> (-158.7794, -153.5158)
  line L5 (-158.7794, -153.5158) -> (-160.3029, -149.0386)
  line L6 (-160.3029, -149.0386) -> (-147.0568, -139.4051)
  arc A0 (-141.7346, -140.2454) -> (-147.0568, -139.4051) centre (-144.8159, -142.4864) ccw
  line L7 (-141.7346, -140.2454) -> (-139.2048, -143.7239)
  line L8 (-139.2048, -143.7239) -> (-141.363, -154.5148)
  arc A1 (-141.363, -154.5148) -> (-126.7925, -176.8522) centre (-122.6829, -158.2508) ccw
  arc A2 (-126.7925, -176.8522) -> (-23.4197, -176.8522) centre (-75.1061, 57.0962) ccw
  arc A3 (-23.4197, -176.8522) -> (-8.8493, -154.5148) centre (-27.5294, -158.2508) ccw
  line L9 (-8.8493, -154.5148) -> (-11.0075, -143.7239)
  line L10 (-11.0075, -143.7239) -> (-8.4776, -140.2454)
  arc A4 (-3.1554, -139.4051) -> (-8.4776, -140.2454) centre (-5.3964, -142.4864) ccw
  line L11 (-3.1554, -139.4051) -> (10.0906, -149.0386)
  line L12 (10.0906, -149.0386) -> (8.5671, -153.5158)
  line L13 (8.5671, -153.5158) -> (10.2135, -154.0761)
  line L14 (10.2135, -154.0761) -> (13.4671, -150.4121)
  line L15 (13.4671, -150.4121) -> (17.879, -137.4466)
  line L16 (17.879, -137.4466) -> (15.8018, -136.844)
  line L17 (15.8018, -136.844) -> (11.0811, -139.4414)
  line L18 (11.0811, -139.4414) -> (10.7402, -140.6166)
  line L19 (10.7402, -140.6166) -> (1.0754, -133.5877)
  arc A5 (0.2351, -128.2655) -> (1.0754, -133.5877) centre (3.3163, -130.5064) ccw
  line L20 (0.2351, -128.2655) -> (6.9957, -118.9696)
  arc A6 (6.9957, -118.9696) -> (8.3661, -111.3412) centre (-0.1939, -113.7407) ccw
  line L21 (8.3661, -111.3412) -> (-23.1898, 1.2301)
  arc A7 (-16.6611, 0.9551) -> (-23.1898, 1.2301) centre (-19.9103, 1.4524) ccw
  arc A8 (-16.6611, 0.9551) -> (-10.3842, -0.0056) centre (-13.5226, 0.4747) ccw
  arc A9 (-10.3842, -0.0056) -> (-29.4342, -0.0197) centre (-19.9103, 1.4524) ccw
  line L22 (-29.4342, -0.0197) -> (2.2518, -113.0551)
  arc A10 (1.8602, -115.2347) -> (2.2518, -113.0551) centre (-0.1939, -113.7407) ccw
  line L23 (1.8602, -115.2347) -> (-17.1252, -141.3396)
  arc A11 (-17.1252, -141.3396) -> (-17.5617, -143.3317) centre (-15.071, -142.8336) ccw
  line L24 (-17.5617, -143.3317) -> (-15.076, -155.7601)
  arc A12 (-24.7896, -170.6518) -> (-15.076, -155.7601) centre (-27.5294, -158.2508) ccw
  arc A13 (-125.4227, -170.6518) -> (-24.7896, -170.6518) centre (-75.1061, 57.0962) ccw
  arc A14 (-135.1363, -155.7601) -> (-125.4227, -170.6518) centre (-122.6829, -158.2508) ccw
  line L25 (-135.1363, -155.7601) -> (-132.6506, -143.3317)
  arc A15 (-132.6506, -143.3317) -> (-133.0871, -141.3396) centre (-135.1413, -142.8336) ccw
  line L26 (-133.0871, -141.3396) -> (-152.0341, -115.2875)
  arc A16 (-152.4258, -113.1086) -> (-152.0341, -115.2875) centre (-149.9799, -113.7935) ccw
  line L27 (-152.4258, -113.1086) -> (-151.4699, -109.6951)
  arc A17 (-151.4699, -109.6951) -> (-21.7483, -130.6442) centre (-45.713, 133.0677) ccw
  arc A18 (-21.7483, -130.6442) -> (-22.4815, -123.2089) centre (-22.86, -127) ccw
  arc A19 (-143.1611, -90.1462) -> (-22.4815, -123.2089) centre (-28.0682, 93.1729) ccw
  arc A20 (-144.8041, -85.892) -> (-143.1611, -90.1462) centre (-141.1353, -86.9194) ccw
  line L28 (-144.8041, -85.892) -> (-120.8502, -0.3539)
  line L29 (-120.8502, -0.3539) -> (-120.7781, -0.0197)
  arc A21 (-120.7781, -0.0197) -> (-139.8281, -0.0056) centre (-130.302, 1.4524) ccw
  arc A22 (-139.8281, -0.0056) -> (-133.5512, 0.9551) centre (-136.6896, 0.4747) ccw
  arc A23 (-127.0318, 1.1197) -> (-133.5512, 0.9551) centre (-130.302, 1.4524) ccw
  line L30 (-127.0318, 1.1197) -> (-158.5406, -111.3962)
  arc A24 (-158.5406, -111.3962) -> (-157.1696, -119.0224) centre (-149.9799, -113.7935) ccw
  line L31 (-157.1696, -119.0224) -> (-150.4473, -128.2655)
  arc A25 (-151.2877, -133.5877) -> (-150.4473, -128.2655) centre (-153.5286, -130.5064) ccw
  line L32 (-151.2877, -133.5877) -> (-160.9524, -140.6166)
  line L33 (-160.9524, -140.6166) -> (-161.2934, -139.4414)
  arc A26 (-126.7925, -176.8522) -> (-23.4197, -176.8522) centre (-75.1061, 57.0962) ccw
  line L34 (-75.1061, -182.4938) -> (-75.1061, -200.66)
  arc A27 (-85.293, -199.9179) -> (-64.9266, -199.9687) centre (-74.93, -127.9586) ccw
  arc A28 (-84.3528, -206.4466) -> (-65.8656, -206.4888) centre (-74.93, -127.9586) ccw
  line L35 (-78.2811, -182.4938) -> (-78.2811, -200.66)
  line L36 (-71.9311, -182.4938) -> (-71.9311, -200.66)
  line L37 (-65.8656, -206.4888) -> (-64.9266, -199.9687)
  line L38 (-84.3467, -206.4888) -> (-85.2856, -199.9687)
  line L39 (-85.2856, -199.9687) -> (-85.293, -199.9179)
  line L40 (-71.9311, -182.4938) -> (-71.9311, -182.2863)
  line L41 (-71.9311, -182.2863) -> (-78.2877, -182.2863)
  line L42 (-78.2877, -182.2863) -> (-78.2811, -182.4938)
  dimension "d56" = 3.175
  dimension "d57" = -3.175
  constraint coincident A1.end A2.start
  constraint coincident A2.end A3.start
  constraint midpoint A26 L34.start
  constraint vertical L34
  constraint coincident L34.end A27
  constraint symmetric L34 A28.end L38.start
  constraint symmetric L34 A27.end L38.end
  constraint concentric A27 A28
  constraint parallel L38 L39
  constraint coincident L38 A28.start
  constraint parallel L36 L40
  constraint perpendicular L40 L41
extrude "Extrude5" add sketch "Sketch14" against normal blind 6.096 separate body contours A2 A26 L34 A27 L35 L42 | A2 A26 L34 A27 L36 L40 | A27 A28 L37 L38 L39 makes body 4
combine "Combine1" operation add target body 2 tool bodies 4
chamfer "Chamfer3" distance 1.27 angle 45 2 edges at (64.9266, 3.048, -199.9687) (85.293, 3.048, -199.9179) on bodies 2
chamfer "Chamfer4" distance 5.08 angle 45 2 edges at (84.3528, 3.048, -206.4466) (65.8656, 3.048, -206.4888) on bodies 2
fillet "Fillet2" radius 6.35 3 edges at (78.2811, 3.048, -182.4938) (78.2818, 3.048, -182.4727) (71.9311, 3.048, -182.4727) on bodies 2
sketch "Sketch15" plane through (159.4134, 0, -115.937) normal (0.808736, 0, -0.588172) x (-0.588172, 0, -0.808736)
  line L0 (3.815, 0) -> (15.2441, 0)
  line L1 (15.2441, 0) -> (15.2441, 6.096)
  line L2 (15.2441, 6.096) -> (3.815, 6.096)
  line L3 (3.815, 6.096) -> (3.815, 0)
  line L4 (18.208, 6.0795) -> (33.02, 6.0795)
  line L5 (33.02, 6.0795) -> (33.02, -0.2705)
  line L6 (33.02, -0.2705) -> (18.208, -0.2705)
  line L7 (18.208, -0.2705) -> (18.208, 6.0795)
  dimension "d63" = 6.35
  constraint horizontal L4
  constraint vertical L5
  constraint horizontal L6
  constraint vertical L7
  measures "d63" distance of L4.start L6.end
extrude "Extrude6" cut sketch "Sketch15" along normal blind 35.56 contours L4 L5 L6 L7 bodies 3
sketch "Sketch16" plane through (0, 0, 0) normal (0, 0, 1) x (1, 0, 0)
  line L0 (79.3054, 6.1492) -> (70.9294, 6.1492)
  line L1 (75.1174, 6.1492) -> (75.1174, 0)
  line L2 (82.7374, 6.3766) -> (67.4974, 6.3766)
  line L3 (67.4974, 6.3766) -> (67.4974, -0.2274)
  line L4 (67.4974, -0.2274) -> (82.7374, -0.2274)
  line L5 (82.7374, -0.2274) -> (82.7374, 6.3766)
  line L6 (82.7374, 6.3766) -> (67.4974, -0.2274) construction
  line L7 (67.4974, 6.3766) -> (82.7374, -0.2274) construction
  point P0 (75.1174, 3.0746)
  dimension "d66" = 15.24
  dimension "d67" = 6.604
  constraint horizontal L0
  constraint midpoint L0 L1.start
  constraint perpendicular L0 L1
  constraint horizontal L2
  constraint perpendicular L2 L3
  constraint parallel L2 L4
  constraint parallel L3 L5
  constraint coincident L6 P0
  constraint coincident L7 P0
  constraint midpoint L1 P0
  measures "d66" distance of L3.end L4.end
  measures "d67" distance of L2.end L3.end
extrude "Extrude7" cut sketch "Sketch16" against normal blind 223.52 bodies 3
ref_plane "WorkPlane1" through (75.1061, 3.048, -98.0512) normal (1, 0, 0) x (0, 0, -1)
mirror "Mirror1" about plane through (75.1061, 3.048, -98.0512) normal (1, 0, 0) of "Extrude6"
hidden bodies 1
